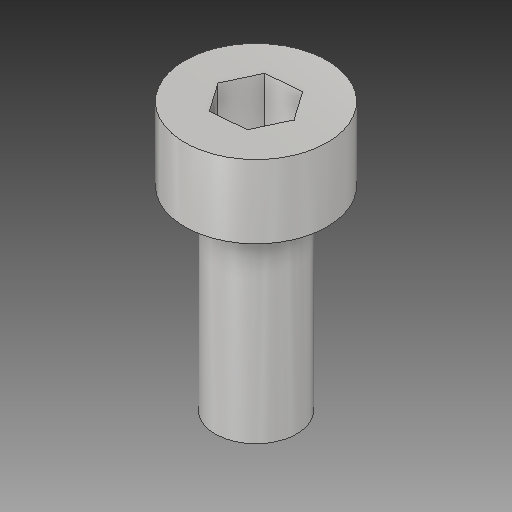
# Autodesk Inventor part: M3_SCREW_8MM
Saved by Autodesk Inventor 2017 (Build 210142000, 142)
## iProperties
Created: 2018-01-04
Part Number: M3_SCREW_8MM
Material: Generic
Document SubType Name: Modeling
Designer: Alex
Density: 1 g/cm^3
Appearance: Aluminum - Polished
d0: 3,350 mm
d1: 8,000 mm
d2: 0,00 deg
d3: 5,850 mm
d4: 3,000 mm
d5: 0,00 deg
d6: 2,500 mm
d7: 1,900 mm
d8: 0,00 deg
screw_m3_A: 3,350 mm
screw_m3_B: 8,000 mm
screw_m3_C: 5,850 mm
screw_m3_D: 3,000 mm
Author: Alex
Autodesk Inventor part; units mm, degrees
ref_plane "YZ Plane" through (0, 0, 0) normal (1, 0, 0) x (0, 1, 0)
ref_plane "XZ Plane" through (0, 0, 0) normal (0, 1, 0) x (-1, 0, 0)
ref_plane "XY Plane" through (0, 0, 0) normal (0, 0, 1) x (1, 0, 0)
sketch "Sketch1" plane through (0, 0, 0) normal (0, 1, 0) x (-1, 0, 0)
  circle A0 centre (0, 0) radius 1.675
  dimension "d0" = 3.35
  constraints: 1 centre point, 1 coincident
  measures "d0" diameter of A0
extrude "Extrusion1" add sketch "Sketch1" along normal blind 8
sketch "Sketch2" plane through (0, 8, 0) normal (0, 1, 0) x (1, 0, 0)
  circle A0 centre (0, 0) radius 1.675 projected
  circle A1 centre (0, 0) radius 2.925
  dimension "d3" = 5.85
  constraints: 1 centre point, 1 coincident
  measures "d3" diameter of A1
extrude "Extrusion2" add sketch "Sketch2" along normal blind 3 contours A0 | A1
sketch "Sketch3" plane through (0, 11, 0) normal (0, 1, 0) x (1, 0, 0)
  line L0 (-0.8268, 1.1831) -> (0.6112, 1.3076)
  line L1 (0.6112, 1.3076) -> (1.438, 0.1244)
  line L2 (1.438, 0.1244) -> (0.8268, -1.1831)
  line L3 (0.8268, -1.1831) -> (-0.6112, -1.3076)
  line L4 (-0.6112, -1.3076) -> (-1.438, -0.1244)
  line L5 (-1.438, -0.1244) -> (-0.8268, 1.1831)
  point P0 (0, 0)
  point P1 (0, 0)
  dimension "d6" = 2.5
  constraints: 12 end point, 1 coincident, 13 other
  measures "d6" distance between parallel lines of L0 L3
extrude "Extrusion3" cut sketch "Sketch3" against normal blind 1.9
equation "\"d0\" = screw_m3_A"
equation "\"d1\" = screw_m3_B"
equation "\"d3\" = screw_m3_C"
equation "\"d4\" = screw_m3_D"
equation "\"screw_m3_B\" = 8"
equation "\"screw_m3_D\" = 3"
equation "\"screw_m3_A\" = 3.35"
equation "\"screw_m3_C\" = 5.85"
body "Solid1"
